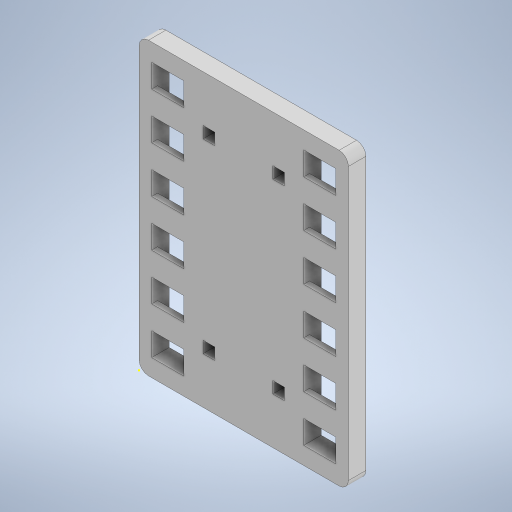
# Autodesk Inventor part: WRO Modell_RC_Auto_3
Saved by Autodesk Inventor 2024 (Build 280153000, 153)
## iProperties
Created: 2025-03-13
Part Number: WRO Modell_RC_Auto_3
Material: Generisch
Document SubType Name: Modeling
Designer: SFZ7-PC
Density: 1 g/cm^3
Appearance: Vorgabe
Author: SFZ7-PC
Autodesk Inventor part; units mm, degrees
ref_plane "YZ Plane" through (0, 0, 0) normal (1, 0, 0) x (0, 1, 0)
ref_plane "XZ Plane" through (0, 0, 0) normal (0, 1, 0) x (-1, 0, 0)
sketch "Skizze1" plane through (0, 0, 0) normal (0, 1, 0) x (-1, 0, 0)
  point P0 (0, 0)
sketch "Skizze2" plane through (0, 0, 0) normal (0, 1, 0) x (-1, 0, 0)
  line L0 (0, 0) -> (-180, 0)
  line L1 (-180, 0) -> (-180, 250)
  line L2 (-180, 250) -> (0, 250)
  line L3 (0, 250) -> (0, 0)
  dimension "d0" = 180
  dimension "d1" = 250
  constraints: 8 end point, 2 parallel, 1 horizontal, 1 perpendicular
  measures "d0" distance of L1.end L2.end
  measures "d1" distance of L0.end L1.end
extrude "Extrusion1" add sketch "Skizze2" along normal blind 15
sketch "Skizze3" plane through (0, 15, 0) normal (0, 1, 0) x (1, 0, 0)
  line L0 (10.7918, -15) -> (38.4358, -15)
  line L1 (38.4358, -15) -> (38.4358, -235)
  line L2 (38.4358, -235) -> (10.7918, -235)
  line L3 (10.7918, -235) -> (10.7918, -15)
  line L4 (0, -250) -> (180, -250) projected
  point P0 (0, 0)
  point P1 (24.6138, -15)
  point P2 (24.6138, -235)
  dimension "d79" = 220
  dimension "d80" = 15
  constraints: 8 end point, 2 midpoint, 2 parallel, 1 horizontal, 1 perpendicular
  measures "d79" distance of point (24.614, -15) point (24.614, -235)
  measures "d80" distance between parallel lines of L2 L4
extrude "Extrusion2" cut sketch "Skizze3" against normal blind 10
sketch "Skizze4" plane through (0, 15, 0) normal (0, 1, 0) x (1, 0, 0)
  line L0 (54.0028, -52.3007) -> (130.0028, -52.3007)
  line L1 (130.0028, -52.3007) -> (130.0028, -96.3007)
  line L2 (130.0028, -96.3007) -> (54.0028, -96.3007)
  line L3 (54.0028, -96.3007) -> (54.0028, -52.3007)
  point P0 (0, 0)
  dimension "d6" = 76
  dimension "d7" = 44
  constraints: 8 end point, 2 parallel, 1 horizontal, 1 perpendicular
  measures "d6" distance of L1.end L2.end
  measures "d7" distance of L0.end L1.end
extrude "Extrusion3" add sketch "Skizze4" along normal blind 5
sketch "Skizze5" plane through (0, 15, 0) normal (0, 1, 0) x (1, 0, 0)
  line L0 (56.8154, -93.8586) -> (61.8154, -93.8586)
  line L1 (61.8154, -93.8586) -> (61.8154, -88.8586)
  line L2 (61.8154, -88.8586) -> (56.8154, -88.8586)
  line L3 (56.8154, -88.8586) -> (56.8154, -93.8586)
  line L4 (56.8154, -55.8667) -> (61.8154, -55.8667)
  line L5 (61.8154, -55.8667) -> (61.8154, -60.8667)
  line L6 (61.8154, -60.8667) -> (56.8154, -60.8667)
  line L7 (56.8154, -60.8667) -> (56.8154, -55.8667)
  point P0 (0, 0)
  dimension "d10" = 5
  dimension "d11" = 5
  dimension "d12" = 5
  constraints: 16 end point, 4 parallel, 2 horizontal, 2 perpendicular
  measures "d10" distance of L2.end L1.end
  measures "d11" distance of L1.end L0.end
  measures "d12" distance of L4.end L5.end
extrude "Extrusion4" add sketch "Skizze5" along normal blind 6 contours L3 L2 L1 L0
sketch "Skizze6" plane through (0, 20, 0) normal (0, 1, 0) x (1, 0, 0)
  line L0 (61.8154, -59.6582) -> (56.8154, -59.6582)
  line L1 (56.8154, -59.6582) -> (56.8154, -54.6582)
  line L2 (56.8154, -54.6582) -> (61.8154, -54.6582)
  line L3 (61.8154, -54.6582) -> (61.8154, -59.6582)
  point P0 (0, 0)
  dimension "d15" = 5
  constraints: 8 end point, 2 parallel, 1 horizontal, 1 perpendicular
  measures "d15" distance of L0.end L1.end
extrude "Extrusion5" add sketch "Skizze6" along normal blind 1
sketch "Skizze7" plane through (0, 20, 0) normal (0, 1, 0) x (1, 0, 0)
  line L0 (121.8231, -54.6582) -> (126.8231, -54.6582)
  line L1 (126.8231, -54.6582) -> (126.8231, -59.6582)
  line L2 (126.8231, -59.6582) -> (121.8231, -59.6582)
  line L3 (121.8231, -59.6582) -> (121.8231, -54.6582)
  point P0 (0, 0)
  dimension "d18" = 5
  constraints: 8 end point, 2 parallel, 1 horizontal, 1 perpendicular
  measures "d18" distance of L1.end L2.end
extrude "Extrusion6" add sketch "Skizze7" along normal blind 1
sketch "Skizze8" plane through (0, 20, 0) normal (0, 1, 0) x (1, 0, 0)
  line L0 (122.1095, -93.6637) -> (127.1095, -93.6637)
  line L1 (127.1095, -93.6637) -> (127.1095, -88.6637)
  line L2 (127.1095, -88.6637) -> (122.1095, -88.6637)
  line L3 (122.1095, -88.6637) -> (122.1095, -93.6637)
  point P0 (0, 0)
  point P1 (124.6095, -93.6637)
  point P2 (124.6095, -88.6637)
  dimension "d21" = 5
  dimension "d22" = 5
  constraints: 8 end point, 2 midpoint, 2 parallel, 1 horizontal, 1 perpendicular
  measures "d21" distance of L2.end L1.end
  measures "d22" distance of point (124.61, -93.664) point (124.61, -88.664)
extrude "Extrusion7" add sketch "Skizze8" along normal blind 1
sketch "Skizze9" plane through (0, 15, 0) normal (0, 1, 0) x (1, 0, 0)
  line L0 (54.0028, -106.6154) -> (124.8609, -106.6154)
  line L1 (124.8609, -106.6154) -> (124.8609, -136.072)
  line L2 (124.8609, -136.072) -> (54.0028, -136.072)
  line L3 (54.0028, -136.072) -> (54.0028, -106.6154)
  line L4 (130.0028, -52.3007) -> (54.0028, -52.3007) projected
  line L5 (54.0028, -96.3007) -> (130.0028, -96.3007) projected
  line L6 (0, -250) -> (180, -250) projected
  point P0 (0, 0)
  point P1 (89.4318, -136.072)
  dimension "d182" = 83.7713
  dimension "d183" = 10.3146
  dimension "d184" = 113.928
  dimension "d185" = 113.928
  constraints: 8 end point, 2 parallel, 1 horizontal, 1 midpoint, 1 perpendicular
  measures "d182" distance between parallel lines of L2 L4
  measures "d183" distance between parallel lines of L0 L5
  measures "d184" distance between parallel lines of L6 L2
  measures "d185" distance from line of L6 point (89.432, -136.072)
extrude "Extrusion8" add sketch "Skizze9" along normal blind 5
sketch "Skizze10" plane through (0, 20, 0) normal (0, 1, 0) x (1, 0, 0)
  line L0 (57.3891, -109.317) -> (59.9809, -109.317)
  line L1 (59.9809, -109.317) -> (59.9809, -134.3091)
  line L2 (59.9809, -134.3091) -> (57.3891, -134.3091)
  line L3 (57.3891, -134.3091) -> (57.3891, -109.317)
  point P0 (0, 0)
  constraints: 8 end point, 2 parallel, 1 horizontal, 1 perpendicular
extrude "Extrusion9" add sketch "Skizze10" along normal blind 1
sketch "Skizze11" plane through (0, 20, 0) normal (0, 1, 0) x (1, 0, 0)
  line L0 (121.6279, -109.6873) -> (119.2213, -109.6873)
  line L1 (119.2213, -109.6873) -> (119.2213, -133.7537)
  line L2 (119.2213, -133.7537) -> (121.6279, -133.7537)
  line L3 (121.6279, -133.7537) -> (121.6279, -109.6873)
  point P0 (0, 0)
  constraints: 8 end point, 2 parallel, 1 horizontal, 1 perpendicular
extrude "Extrusion10" add sketch "Skizze11" along normal blind 1
sketch "Skizze14" plane through (0, 5, 0) normal (0, 1, 0) x (1, 0, 0)
  line L0 (10.7918, -235) -> (10.7918, -15) projected
  line L1 (38.4358, -15) -> (38.4358, -235) projected
  line L2 (10.7918, -15) -> (38.4358, -15)
  line L3 (38.4358, -15) -> (38.4358, -35)
  line L4 (38.4358, -35) -> (10.7918, -35)
  line L5 (10.7918, -35) -> (10.7918, -15)
  line L6 (10.7918, -55) -> (38.4358, -55)
  line L7 (38.4358, -55) -> (38.4358, -75)
  line L8 (38.4358, -75) -> (10.7918, -75)
  line L9 (10.7918, -75) -> (10.7918, -55)
  line L10 (10.7918, -95) -> (38.4358, -95)
  line L11 (38.4358, -95) -> (38.4358, -115)
  line L12 (38.4358, -115) -> (10.7918, -115)
  line L13 (10.7918, -115) -> (10.7918, -95)
  line L14 (10.7918, -135) -> (38.4358, -135)
  line L15 (38.4358, -135) -> (38.4358, -155)
  line L16 (38.4358, -155) -> (10.7918, -155)
  line L17 (10.7918, -155) -> (10.7918, -135)
  line L18 (10.7918, -175) -> (38.4358, -175)
  line L19 (38.4358, -175) -> (38.4358, -195)
  line L20 (38.4358, -195) -> (10.7918, -195)
  line L21 (10.7918, -195) -> (10.7918, -175)
  line L22 (10.7918, -215) -> (38.4358, -215)
  line L23 (38.4358, -215) -> (38.4358, -235)
  line L24 (38.4358, -235) -> (10.7918, -235)
  line L25 (10.7918, -235) -> (10.7918, -215)
  point P0 (0, 0)
  point P1 (24.6138, -55)
  point P2 (24.6138, -35)
  point P3 (24.6138, -95)
  point P4 (24.6138, -135)
  point P5 (24.6138, -175)
  point P6 (24.6138, -155)
  point P7 (24.6138, -215)
  point P8 (24.6138, -195)
  point P9 (10.7918, -235)
  point P10 (38.4358, -215)
  point P11 (10.7918, -195)
  point P12 (38.4358, -175)
  point P13 (10.7918, -155)
  point P14 (38.4358, -135)
  point P15 (10.7918, -115)
  point P16 (38.4358, -95)
  point P17 (10.7918, -75)
  point P18 (38.4358, -55)
  point P19 (10.7918, -55)
  point P20 (10.7918, -35)
  dimension "d42" = 20
  dimension "d43" = 20
  dimension "d44" = 20
  dimension "d45" = 20
  dimension "d46" = 20
  dimension "d47" = 20
  dimension "d48" = 20
  dimension "d49" = 20
  dimension "d50" = 20
  dimension "d51" = 20
  dimension "d52" = 20
  constraints: 48 end point, 12 parallel, 11 point on line, 8 midpoint, 6 horizontal, 6 perpendicular
  measures "d42" distance of L2.end L3.end
  measures "d43" distance of L6.end L7.end
  measures "d44" distance of point (24.614, -55) point (24.614, -35)
  measures "d45" distance of L10.end L11.end
  measures "d46" distance of L14.end L15.end
  measures "d47" distance from line of point (24.614, -95) L8
  measures "d48" distance from line of point (24.614, -135) L12
  measures "d49" distance of L18.end L19.end
  measures "d50" distance of L22.end L23.end
  measures "d51" distance of point (24.614, -175) point (24.614, -155)
  measures "d52" distance of point (24.614, -215) point (24.614, -195)
extrude "Extrusion12" cut sketch "Skizze14" against normal blind 20 contours L0 L22 L1 L24 | L0 L18 L1 L20 | L0 L14 L1 L16 | L0 L10 L1 L12 | L0 L6 L1 L8 | L0 L2 L1 L4
ref_plane "Arbeitsebene1" through (90, 0, 250) normal (1, 0, 0) x (0, 0, -1)
mirror "Spiegeln1" about plane through (90, 0, 250) normal (1, 0, 0) of "Extrusion12"
mirror "Spiegeln2" about plane through (90, 0, 250) normal (1, 0, 0) of "Extrusion2"
sketch "Skizze15" plane through (0, 15, 0) normal (0, 1, 0) x (1, 0, 0)
  line L0 (55, -210) -> (65, -210)
  line L1 (65, -210) -> (65, -200)
  line L2 (65, -200) -> (55, -200)
  line L3 (55, -200) -> (55, -210)
  line L4 (115, -210) -> (125, -210)
  line L5 (125, -210) -> (125, -200)
  line L6 (125, -200) -> (115, -200)
  line L7 (115, -200) -> (115, -210)
  line L8 (0, -250) -> (180, -250) projected
  line L9 (55, -50) -> (65, -50)
  line L10 (65, -50) -> (65, -40)
  line L11 (65, -40) -> (55, -40)
  line L12 (55, -40) -> (55, -50)
  line L13 (115, -50) -> (125, -50)
  line L14 (125, -50) -> (125, -40)
  line L15 (125, -40) -> (115, -40)
  line L16 (115, -40) -> (115, -50)
  line L17 (0, 0) -> (0, -250) projected
  line L18 (180, -250) -> (180, 0) projected
  line L19 (180, 0) -> (0, 0) projected
  point P0 (120, -210)
  point P1 (60, -50)
  point P2 (120, -50)
  point P3 (55, -205)
  point P4 (125, -205)
  point P5 (55, -45)
  point P6 (125, -45)
  point P7 (60, -210)
  point P8 (60, -40)
  point P9 (120, -40)
  dimension "d56" = 10
  dimension "d57" = 10
  dimension "d58" = 10
  dimension "d59" = 10
  dimension "d60" = 40
  dimension "d61" = 10
  dimension "d62" = 10
  dimension "d63" = 10
  dimension "d64" = 10
  dimension "d72" = 55
  dimension "d73" = 55
  dimension "d74" = 55
  dimension "d75" = 55
  dimension "d76" = 40
  dimension "d77" = 40
  dimension "d78" = 40
  constraints: 32 end point, 10 midpoint, 8 parallel, 4 horizontal, 4 perpendicular
  measures "d56" distance of L2.end L1.end
  measures "d57" distance of L1.end L0.end
  measures "d58" distance of L6.end L5.end
  measures "d59" distance of L5.end L4.end
  measures "d60" distance from line of point (120, -210) L8
  measures "d61" distance of L11.end L10.end
  measures "d62" distance of L10.end L9.end
  measures "d63" distance of L15.end L14.end
  measures "d64" distance of L14.end L13.end
  measures "d72" distance from line of L17 point (55, -205)
  measures "d73" distance from line of L18 point (125, -205)
  measures "d74" distance from line of point (55, -45) L17
  measures "d75" distance from line of point (125, -45) L18
  measures "d76" distance from line of point (60, -210) L8
  measures "d77" distance from line of L19 point (60, -40)
  measures "d78" distance from line of L19 point (120, -40)
extrude "Extrusion13" cut sketch "Skizze15" against normal blind 20 contours L3 L2 L1 L0 | L7 L6 L5 L4 | L12 L11 L10 L9 | L16 L15 L14 L13
fillet "Rundung9" radius 8 4 edges at (180, 7.5, 250) (180, 7.5, 0) (0, 7.5, 0) (0, 7.5, 250)
